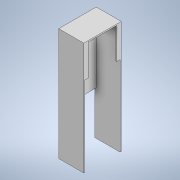
# Autodesk Inventor part: Soporte_camara
Saved by Autodesk Inventor 2020 (Build 240168000, 168)
## iProperties
Created: 2023-03-22
Part Number: Soporte_camara
Material: Generic
Document SubType Name: Modeling
Designer: semon
Density: 1 g/cm^3
Appearance: Default
Author: semon
Autodesk Inventor part; units mm, degrees
ref_plane "YZ Plane" through (0, 0, 0) normal (1, 0, 0) x (0, 1, 0)
ref_plane "XZ Plane" through (0, 0, 0) normal (0, 1, 0) x (-1, 0, 0)
ref_plane "XY Plane" through (0, 0, 0) normal (0, 0, 1) x (1, 0, 0)
sketch "Sketch1" plane through (0, 0, 0) normal (0, 1, 0) x (-1, 0, 0)
  line L0 (0, -28) -> (38, -28)
  line L1 (38, -28) -> (38, 28)
  line L2 (38, 28) -> (0, 28)
  line L3 (0, 28) -> (0, -28) construction
  line L4 (0, 30) -> (40, 30)
  line L5 (40, 30) -> (40, -30)
  line L6 (40, -30) -> (0, -30)
  line L7 (0, 30) -> (0, 28)
  line L8 (0, -28) -> (0, -30)
  point P0 (0, 0)
  point P1 (0, 0)
  dimension "d0" = 40
  dimension "d1" = 60
  dimension "d2" = 2
  dimension "d3" = 38
  constraints: 18 end point, 4 equal length, 2 horizontal, 2 perpendicular, 1 coincident, 1 collinear, 1 midpoint, 1 vertical
  measures "d0" distance of L5.end L6.end
  measures "d1" distance of L4.end L5.end
  measures "d2" distance between parallel lines of L6 L0
  measures "d3" distance of L1.end L2.end
extrude "Extrusion1" add sketch "Sketch1" along normal blind 180
sketch "Sketch2" plane through (0, 180, 0) normal (0, 1, 0) x (1, 0, 0)
  line L0 (-38, 28) -> (0, 28) projected
  line L1 (0, -30) -> (0, -28) projected
  line L2 (-38, 28) -> (0, 28)
  line L3 (0, 28) -> (0, -28)
  line L4 (0, -28) -> (-38, -28)
  line L5 (-38, -28) -> (-38, 28)
  point P0 (0, 0)
  constraints: 8 end point, 2 parallel, 1 horizontal, 1 perpendicular
extrude "Extrusion2" add sketch "Sketch2" against normal blind 2
sketch "Sketch3" plane through (-38, 0, -28) normal (0, 0, 1) x (1, 0, 0)
  line L0 (38, 178) -> (36, 178)
  line L1 (36, 178) -> (36, 128)
  line L2 (36, 128) -> (38, 128)
  line L3 (38, 128) -> (38, 178)
  point P0 (38, 0)
  dimension "d8" = 2
  dimension "d9" = 50
  constraints: 8 end point, 2 parallel, 1 horizontal, 1 perpendicular
  measures "d8" distance of L2.end L1.end
  measures "d9" distance of L0.end L1.end
extrude "Extrusion3" add sketch "Sketch3" along normal blind 5
mirror "Mirror1" about plane through (0, 0, 0) normal (0, 0, 1) of "Extrusion3"
sketch "Sketch4" plane through (-38, 0, 28) normal (1, 0, 0) x (0, 0, -1)
  line L0 (0, 0) -> (56, 0) projected
  line L1 (56, 0) -> (56, 178) projected
  line L2 (0, 0) -> (56, 0)
  line L3 (56, 0) -> (56, 70)
  line L4 (56, 70) -> (0, 70)
  line L5 (0, 70) -> (0, 0)
  point P0 (28, 0)
  dimension "d12" = 70
  constraints: 8 end point, 2 parallel, 1 horizontal, 1 perpendicular, 1 point on line
  measures "d12" distance of L3.end L2.end
extrude "Extrusion4" cut sketch "Sketch4" against normal blind 5
body "Solid1"
